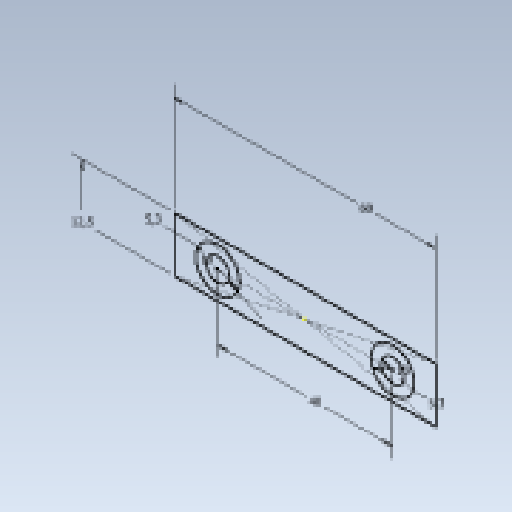
# Autodesk Inventor part: Soporte Switch Y
Saved by Autodesk Inventor 2024.2 (Build 282272000, 272)
## iProperties
Created: 2024-05-31
Part Number: Soporte Switch Y
Material: Generic
Document SubType Name: Modeling
Designer: jp.reyesf
Density: 1 g/cm^3
Appearance: Default
Author: jp.reyesf
Autodesk Inventor part; units mm, degrees
ref_plane "YZ Plane" through (0, 0, 0) normal (1, 0, 0) x (0, 1, 0)
ref_plane "XZ Plane" through (0, 0, 0) normal (0, 1, 0) x (-1, 0, 0)
ref_plane "XY Plane" through (0, 0, 0) normal (0, 0, 1) x (1, 0, 0)
sketch "Sketch1" plane through (0, 0, 0) normal (0, 0, 1) x (1, 0, 0)
  line L0 (-40, -6.25) -> (40, -6.25)
  line L1 (40, -6.25) -> (40, 6.25)
  line L2 (40, 6.25) -> (-40, 6.25)
  line L3 (-40, 6.25) -> (-40, -6.25)
  line L4 (-40, -6.25) -> (40, 6.25) construction
  line L5 (40, -6.25) -> (-40, 6.25) construction
  line L6 (-30, 0) -> (30, 0) construction
  circle A0 centre (-30, 0) radius 2.65
  circle A1 centre (30, 0) radius 2.65
  circle A2 centre (-30, 0) radius 5
  circle A3 centre (30, 0) radius 5
  line L7 (-40, 6.25) -> (-37, 6.25)
  line L8 (-37, 6.25) -> (-37, -6.25)
  line L9 (-37, -6.25) -> (-40, -6.25)
  line L10 (-40, -6.25) -> (-40, 6.25)
  line L11 (40, -6.25) -> (37, -6.25)
  line L12 (37, -6.25) -> (37, 6.25)
  line L13 (37, 6.25) -> (40, 6.25)
  line L14 (40, 6.25) -> (40, -6.25)
  line L15 (-40, 6.25) -> (40, 6.25)
  line L16 (40, 6.25) -> (40, 3.25)
  line L17 (40, 3.25) -> (-40, 3.25)
  line L18 (-40, 3.25) -> (-40, 6.25)
  point P0 (0, 0)
  point P1 (-37, 3.25)
  point P2 (-33.7997, 3.25)
  point P3 (-26.2003, 3.25)
  point P4 (26.2003, 3.25)
  point P5 (33.7997, 3.25)
  point P6 (37, 3.25)
  dimension "d0" = 80
  dimension "d1" = 12.5
  dimension "d2" = 60
  dimension "d3" = 5.3
  dimension "d4" = 5.3
  dimension "d5" = 10
  dimension "d6" = 10
  dimension "d9" = 3
  dimension "d10" = 3
  dimension "d11" = 3
  constraints: 38 end point, 8 parallel, 5 horizontal, 4 centre point, 4 coincident, 4 perpendicular, 3 midpoint, 3 point on line
  measures "d0" distance between parallel lines of L1 L3
  measures "d1" distance between parallel lines of L0 L2
  measures "d2" distance of L6.start L6.end
  measures "d3" diameter of A0
  measures "d4" diameter of A1
  measures "d5" diameter of A2
  measures "d6" diameter of A3
  measures "d9" distance between parallel lines of L3 L8
  measures "d10" distance between parallel lines of L1 L12
  measures "d11" distance between parallel lines of L2 L17
extrude "Extrusion1" add sketch "Sketch1" along normal blind 3
extrude "Extrusion2" add sketch "Sketch1" along normal blind 60 contours L3 L17 L8 L0 | L3 L2 L8 L17 | L12 L17 L1 L0 | L8 L2 L12 L17 A3 A2 | L12 L2 L1 L17
chamfer "Chamfer1" distance 9.49 angle 45 2 edges at (-38.5, -6.25, 60) (38.5, -6.25, 60)
sketch "Sketch2" plane through (-26.2003, 3.25, 3) normal (0, -1, 0) x (1, 0, 0)
  line L0 (11.2003, 27) -> (11.2003, 47) construction
  line L1 (14.5003, 27) -> (14.5003, 47)
  line L2 (7.9003, 47) -> (7.9003, 27)
  arc A0 (7.9003, 27) -> (14.5003, 27) centre (11.2003, 27) ccw
  arc A1 (14.5003, 47) -> (7.9003, 47) centre (11.2003, 47) ccw
  line L3 (41.2003, 27) -> (41.2003, 47) construction
  line L4 (37.9003, 27) -> (37.9003, 47)
  line L5 (44.5003, 47) -> (44.5003, 27)
  arc A2 (37.9003, 27) -> (44.5003, 27) centre (41.2003, 27) ccw
  arc A3 (44.5003, 47) -> (37.9003, 47) centre (41.2003, 47) ccw
  line L6 (11.2003, 37) -> (41.2003, 37) construction
  line L7 (26.2003, 37) -> (26.2003, 57) construction
  line L8 (0, 57) -> (52.4007, 57) projected
  line L9 (2.9003, 27) -> (49.5003, 27)
  line L10 (49.5003, 27) -> (49.5003, 77)
  line L11 (49.5003, 77) -> (2.9003, 77)
  line L12 (2.9003, 77) -> (2.9003, 27)
  line L13 (26.2003, 27) -> (26.2003, 37) construction
  circle A4 centre (11.2003, 37) radius 3.3
  circle A5 centre (41.2003, 37) radius 3.3
  point P0 (26.2003, -3)
  dimension "d17" = 30
  dimension "d18" = 20
  dimension "d19" = 20
  dimension "d20" = 3.3
  dimension "d21" = 5
  dimension "d29" = 20
  dimension "d30" = 10
  constraints: 30 end point, 8 point on circle, 8 tangent, 6 centre point, 6 parallel, 5 midpoint, 3 equal radius, 3 perpendicular, 2 coincident, 2 vertical, 1 horizontal
  measures "d17" distance of L6.start L6.end
  measures "d18" distance of L0.start L0.end
  measures "d19" distance of L7.start L7.end
  measures "d20" radius of A1
  measures "d21" distance between parallel lines of L12 L2
  measures "d29" distance between parallel lines of L11 L8
  measures "d30" distance from line of L9 L6.start
extrude "Extrusion3" cut sketch "Sketch2" against normal through all contours L9 L2 A4 L1 | A0 L9 | A4 L2 A1 L1 | A4 | L9 A2 | L4 A5 L5 L9 | L4 A3 L5 A5 | A5
extrude "Extrusion4" add sketch "Sketch2" along normal blind 5 separate body contours L9 L2 A4 L1 | L1 A1 L2 L9 L12 L8 L10 L5 A3 L4 | A4 L2 A1 L1 | L4 A5 L5 L9 | L4 A3 L5 A5 | L12 L11 L10 L8
sketch "Sketch3" plane through (-26.2003, -1.75, 3) normal (0, -1, 0) x (1, 0, 0)
  line L0 (5.9503, 60.9) -> (5.9503, 77)
  line L1 (5.9503, 77) -> (46.4503, 77)
  line L2 (46.4503, 77) -> (46.4503, 60.9)
  line L3 (46.4503, 60.9) -> (5.9503, 60.9)
  line L4 (24.2503, 74.35) -> (43.3503, 74.35) construction
  circle A0 centre (24.2503, 74.35) radius 1.5
  circle A1 centre (43.3503, 74.35) radius 1.5
  line L5 (49.5003, 77) -> (2.9003, 77) projected
  line L6 (26.2003, 77) -> (26.2003, 77)
  point P0 (26.2003, -3)
  dimension "d31" = 3
  dimension "d32" = 19.1
  dimension "d34" = 2.65
  dimension "d35" = 16.1
  dimension "d36" = 40.5
  dimension "d37" = 0
  dimension "d40" = 3.1
  constraints: 12 end point, 3 parallel, 2 centre point, 2 coincident, 2 midpoint, 2 perpendicular, 1 equal radius
  measures "d31" diameter of A0
  measures "d32" distance of L4.start L4.end
  measures "d34" distance between parallel lines of L1 L4
  measures "d35" distance of L0.start L0.end
  measures "d36" distance between parallel lines of L0 L2
  measures "d37" distance of L6.start L6.end
  measures "d40" distance from line of L2 L4.end
extrude "Extrusion5" cut sketch "Sketch3" against normal through all contours A0 | A1 bodies 2
body "Solid1"
body "Solid2"
